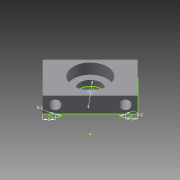
# Autodesk Inventor part: bearing_holder_corner
Saved by Autodesk Inventor 2015 (Build 190159000, 159)
## iProperties
Created: 2017-12-15
Part Number: bearing_holder_corner
Material: Generic
Document SubType Name: Modeling
Designer: Anshul
Density: 1 g/cm^3
Appearance: Default
Author: Anshul
Autodesk Inventor part; units mm, degrees
ref_plane "YZ Plane" through (0, 0, 0) normal (1, 0, 0) x (0, 1, 0)
ref_plane "XZ Plane" through (0, 0, 0) normal (0, 1, 0) x (-1, 0, 0)
ref_plane "XY Plane" through (0, 0, 0) normal (0, 0, 1) x (1, 0, 0)
sketch "Sketch1" plane through (0, 0, 0) normal (0, 1, 0) x (-1, 0, 0)
  line L0 (20, 0) -> (0, -20)
  circle A0 centre (19.5459, -19.5459) radius 9.65
  circle A1 centre (0, -20) radius 2.6
  circle A2 centre (20, 0) radius 2.6
  line L1 (18.1615, -1.8385) -> (27.7075, -11.3844)
  line L2 (27.7075, -11.3844) -> (26.3695, -12.7224)
  line L3 (1.8385, -18.1615) -> (11.3844, -27.7075)
  line L4 (11.3844, -27.7075) -> (12.7224, -26.3695)
  circle A3 centre (19.5459, -19.5459) radius 11.5421
  line L5 (27.7075, -27.7075) -> (19.5459, -35.869)
  line L6 (19.5459, -35.869) -> (11.3844, -27.7075)
  line L7 (27.7075, -27.7075) -> (35.869, -19.5459)
  line L8 (35.869, -19.5459) -> (27.7075, -11.3844)
  circle A4 centre (19.5459, -19.5459) radius 6
  line L9 (20, 0) -> (23.5355, 3.5355)
  line L10 (23.5355, 3.5355) -> (41.243, -14.1719)
  line L11 (35.869, -19.5459) -> (41.243, -14.1719)
  line L12 (0, -20) -> (-3.5355, -23.5355)
  line L13 (-3.5355, -23.5355) -> (14.1719, -41.243)
  line L14 (14.1719, -41.243) -> (19.5459, -35.869)
  line L15 (18.1615, -1.8385) -> (23.5355, 3.5355)
  line L16 (41.243, -14.1719) -> (35.869, -19.5459)
  line L17 (35.869, -19.5459) -> (19.5459, -35.869)
  line L18 (1.8385, -18.1615) -> (-3.5355, -23.5355)
  line L19 (18.1615, -1.8385) -> (1.8385, -18.1615)
  point P0 (0, 0)
  dimension "d6" = 5.2
  dimension "d7" = 5.2
  dimension "d9" = 5
  dimension "d10" = 5
  dimension "d15" = 19.3
  constraints: 40 end point, 7 collinear, 5 perpendicular, 4 coincident, 4 point on circle, 4 point on line, 3 centre point, 3 tangent, 1 parallel, 8 other
  measures "d9" distance of L9.start L9.end
  measures "d10" distance of L12.start L12.end
  measures "d15" diameter of A0
extrude "Extrusion1" add sketch "Sketch1" along normal blind 3 contours A0
extrude "Extrusion2" add sketch "Sketch1" along normal blind 9 contours L9 A2 L0 | L1 A3 L3 L0 | A2 L9 L10 L11 L8 L1 | A1 L12 L0 | L3 L6 L14 L13 L12 A1 | A3 L4 A0 L2 | L8 L7 A3 | L2 A0 L4 A3 | A3 L5 L6 picked at (18.9343, -1.3518) picked at (1.1684, -21.264)
sketch "Sketch2" plane through (-14.1719, 0, -41.243) normal (-0.7071, 0, -0.7071) x (-0.7071, 0, 0.7071)
  line L0 (38.2843, 0) -> (38.2843, 4.5)
  line L1 (38.2843, 0) -> (38.2843, 9) projected
  line L2 (0, 0) -> (0, 4.5)
  line L3 (0, 0) -> (0, 9) projected
  line L4 (0, 4.5) -> (5, 4.5)
  line L5 (38.2843, 4.5) -> (33.2843, 4.5)
  circle A0 centre (33.2843, 4.5) radius 2.6
  circle A1 centre (5, 4.5) radius 2.6
  point P0 (19.1421, 0)
  dimension "d16" = 5
  dimension "d17" = 5
  dimension "d18" = 5.2
  dimension "d19" = 5.2
  constraints: 8 end point, 2 centre point, 2 coincident, 2 midpoint, 1 perpendicular, 1 point on line
  measures "d16" distance of L2.end L4.end
  measures "d17" distance of L0.end L5.end
  measures "d18" diameter of A0
  measures "d19" diameter of A1
extrude "Extrusion3" cut sketch "Sketch2" against normal blind 30
body "Solid1"
